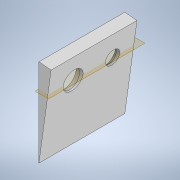
# Autodesk Inventor part: twoPipeCover02
Saved by Autodesk Inventor 2021.1 (Build 251245000, 245)
## iProperties
Created: 2020-07-06
Part Number: twoPipeCover02
Material: Generic
Document SubType Name: Modeling
Designer: robst
Density: 1 g/cm^3
Appearance: Default
Author: robst
Autodesk Inventor part; units mm, degrees
ref_plane "YZ Plane" through (0, 0, 0) normal (1, 0, 0) x (0, 1, 0)
sketch "Sketch1" plane through (0, 0, 0) normal (0, 0, 1) x (1, 0, 0)
  line L0 (0, 0) -> (14.2789, 101.6)
  line L1 (14.2789, 101.6) -> (0, 101.6)
  line L2 (0, 101.6) -> (0, 0)
  dimension "d0" = 101.6
  dimension "d1" = 8
  dimension "d2" = 14.279
  constraints: 6 end point, 1 horizontal, 1 vertical
  measures "d0" distance from line of L0.start L1
  measures "d1" angle of L0 L2
  measures "d2" distance of L0.end L1.end
extrude "MainStructure" add sketch "Sketch1" along normal mid plane 78.74
sketch "Sketch2" plane through (0, 0, 39.37) normal (-1, 0, 0) x (0, 0, 1)
  line L0 (-78.74, 101.6) -> (0, 101.6) projected
  line L1 (-39.37, 101.6) -> (-39.37, 0) construction
  circle A0 centre (-62.23, 73.66) radius 8.255
  circle A1 centre (-16.51, 73.66) radius 11.43
  dimension "d31" = 27.94
  dimension "d32" = 27.94
  dimension "d33" = 22.86
  dimension "d34" = 22.86
  dimension "leftHole" = 22.86
  dimension "rightHole" = 16.51
  constraints: 2 centre point, 2 end point, 1 midpoint, 1 vertical
  measures "d31" distance from line of A0.centre L0
  measures "d32" distance from line of A1.centre L0
  measures "d33" distance from line of A0.centre L1
  measures "d34" distance from line of A1.centre L1
  measures "leftHole" diameter of A1
  measures "rightHole" diameter of A0
extrude "PipeHole" cut sketch "Sketch2" against normal through all
sketch "Sketch6" plane through (0, 0, 0) normal (0, 0, 1) x (1, 0, 0)
  line L0 (0, 101.6) -> (14.2789, 101.6) projected
  line L1 (0, 0) -> (0, 101.6) projected
  line L2 (14.2789, 101.6) -> (0, 0) projected
  line L3 (0, 101.6) -> (14.1055, 100.3659)
  line L4 (14.1055, 100.3659) -> (14.2789, 101.6)
  line L5 (14.2789, 101.6) -> (0, 101.6)
  dimension "d18" = 5
  constraints: 6 end point, 1 collinear, 1 point on line
  measures "d18" angle of L3 L0
extrude "AngleForTopRelief" cut sketch "Sketch6" along normal through all both and the other way through all contours L0 L2 L3
sketch "Sketch7" plane through (0, 0, -39.37) normal (-1, 0, 0) x (0, 0, 1)
  line L0 (0, 0) -> (0, 101.6) construction
  line L1 (0, 50.8) -> (78.74, 50.8) construction
  line L2 (78.74, 0) -> (78.74, 100.3659) construction
  line L3 (0, 0) -> (78.74, 0) projected
  spline S0 degree 2 poles (20.3251, 48.3506) (20.3251, 47.4037) (19.6047, 45.9526) (19.0078, 45.4792) knots 0 0 0 1 2 2 2
  spline S1 degree 2 poles (19.0078, 45.4792) (18.2874, 44.9234) (16.651, 44.45) (15.3542, 44.45) knots 0 0 0 1 2 2 2
  line L4 (15.3542, 44.45) -> (11.711, 44.45)
  line L5 (11.711, 44.45) -> (11.711, 57.15)
  line L6 (11.711, 57.15) -> (15.0764, 57.15)
  spline S2 degree 2 poles (15.0764, 57.15) (16.4349, 57.15) (17.7934, 56.975) (18.4109, 56.6354) knots 0 0 0 1 2 2 2
  spline S3 degree 2 poles (18.4109, 56.6354) (19.1004, 56.2752) (19.7282, 55.0917) (19.7282, 54.2889) knots 0 0 0 1 2 2 2
  spline S4 degree 2 poles (19.7282, 54.2889) (19.7282, 53.3935) (18.7814, 51.9733) (17.9478, 51.5719) knots 0 0 0 1 2 2 2
  line L7 (17.9478, 51.5719) -> (17.9478, 51.5101)
  spline S5 degree 2 poles (17.9478, 51.5101) (19.0798, 51.2014) (20.3251, 49.565) (20.3251, 48.3506) knots 0 0 0 1 2 2 2
  spline S6 degree 2 poles (18.5653, 48.2785) (18.5653, 48.9989) (18.1536, 49.9252) (17.5361, 50.2545) knots 0 0 0 1 2 2 2
  spline S7 degree 2 poles (17.5361, 50.2545) (17.1347, 50.4604) (16.1879, 50.5839) (15.3131, 50.5839) knots 0 0 0 1 2 2 2
  line L8 (15.3131, 50.5839) -> (13.3988, 50.5839)
  line L9 (13.3988, 50.5839) -> (13.3988, 45.8908)
  line L10 (13.3988, 45.8908) -> (14.7676, 45.8908)
  spline S8 degree 2 poles (14.7676, 45.8908) (15.8791, 45.8908) (17.1553, 46.0967) (17.6493, 46.426) knots 0 0 0 1 2 2 2
  spline S9 degree 2 poles (17.6493, 46.426) (18.1227, 46.7656) (18.5653, 47.6096) (18.5653, 48.2785) knots 0 0 0 1 2 2 2
  spline S10 degree 2 poles (17.9683, 54.0522) (17.9683, 54.505) (17.6596, 55.1843) (17.32, 55.3798) knots 0 0 0 1 2 2 2
  spline S11 degree 2 poles (17.32, 55.3798) (16.9083, 55.6062) (15.91, 55.7092) (15.0146, 55.7092) knots 0 0 0 1 2 2 2
  line L11 (15.0146, 55.7092) -> (13.3988, 55.7092)
  line L12 (13.3988, 55.7092) -> (13.3988, 51.9938)
  line L13 (13.3988, 51.9938) -> (15.3131, 51.9938)
  spline S12 degree 2 poles (15.3131, 51.9938) (16.1055, 51.9938) (16.8568, 52.1585) (17.2582, 52.4158) knots 0 0 0 1 2 2 2
  spline S13 degree 2 poles (17.2582, 52.4158) (17.6493, 52.6628) (17.9683, 53.4553) (17.9683, 54.0522) knots 0 0 0 1 2 2 2
  line L14 (26.0885, 44.45) -> (30.3699, 57.15)
  line L15 (30.3699, 57.15) -> (32.4488, 57.15)
  line L16 (32.4488, 57.15) -> (36.7302, 44.45)
  line L17 (36.7302, 44.45) -> (34.9497, 44.45)
  line L18 (34.9497, 44.45) -> (33.797, 48.0006)
  line L19 (33.797, 48.0006) -> (28.9496, 48.0006)
  line L20 (28.9496, 48.0006) -> (27.7969, 44.45)
  line L21 (27.7969, 44.45) -> (26.0885, 44.45)
  line L22 (33.3339, 49.4415) -> (31.3682, 55.421)
  line L23 (31.3682, 55.421) -> (29.4127, 49.4415)
  line L24 (29.4127, 49.4415) -> (33.3339, 49.4415)
  spline S14 degree 2 poles (48.5142, 44.2236) (47.2792, 44.2236) (45.19, 45.0572) (44.4284, 45.8908) knots 0 0 0 1 2 2 2
  spline S15 degree 2 poles (44.4284, 45.8908) (43.6668, 46.7142) (42.8332, 49.1842) (42.8332, 50.7897) knots 0 0 0 1 2 2 2
  spline S16 degree 2 poles (42.8332, 50.7897) (42.8332, 52.3849) (43.6462, 54.752) (44.4181, 55.6268) knots 0 0 0 1 2 2 2
  spline S17 degree 2 poles (44.4181, 55.6268) (45.1797, 56.481) (47.2586, 57.3764) (48.5451, 57.3764) knots 0 0 0 1 2 2 2
  spline S18 degree 2 poles (48.5451, 57.3764) (49.1832, 57.3764) (50.305, 57.1912) (50.7784, 57.0471) knots 0 0 0 1 2 2 2
  spline S19 degree 2 poles (50.7784, 57.0471) (51.1901, 56.9133) (52.0443, 56.5325) (52.4662, 56.3061) knots 0 0 0 1 2 2 2
  line L25 (52.4662, 56.3061) -> (52.4662, 54.2683)
  line L26 (52.4662, 54.2683) -> (52.3324, 54.2683)
  spline S20 degree 2 poles (52.3324, 54.2683) (52.106, 54.4741) (51.4062, 55.0505) (50.9019, 55.3284) knots 0 0 0 1 2 2 2
  spline S21 degree 2 poles (50.9019, 55.3284) (50.4182, 55.5959) (49.2758, 55.9356) (48.5348, 55.9356) knots 0 0 0 1 2 2 2
  spline S22 degree 2 poles (48.5348, 55.9356) (47.7217, 55.9356) (46.2706, 55.2666) (45.7251, 54.6285) knots 0 0 0 1 2 2 2
  spline S23 degree 2 poles (45.7251, 54.6285) (45.19, 53.9801) (44.5931, 52.0144) (44.5931, 50.7897) knots 0 0 0 1 2 2 2
  spline S24 degree 2 poles (44.5931, 50.7897) (44.5931, 49.4827) (45.2209, 47.5993) (45.7663, 46.9509) knots 0 0 0 1 2 2 2
  spline S25 degree 2 poles (45.7663, 46.9509) (46.3015, 46.3231) (47.732, 45.685) (48.5348, 45.685) knots 0 0 0 1 2 2 2
  spline S26 degree 2 poles (48.5348, 45.685) (49.2655, 45.685) (50.5108, 46.0452) (50.9945, 46.3128) knots 0 0 0 1 2 2 2
  spline S27 degree 2 poles (50.9945, 46.3128) (51.4576, 46.5804) (52.1472, 47.1361) (52.3427, 47.3317) knots 0 0 0 1 2 2 2
  line L27 (52.3427, 47.3317) -> (52.4662, 47.3317)
  line L28 (52.4662, 47.3317) -> (52.4662, 45.3145)
  spline S28 degree 2 poles (52.4662, 45.3145) (52.0443, 45.119) (51.3033, 44.7588) (50.7784, 44.5941) knots 0 0 0 1 2 2 2
  spline S29 degree 2 poles (50.7784, 44.5941) (50.2226, 44.4088) (49.2758, 44.2236) (48.5142, 44.2236) knots 0 0 0 1 2 2 2
  line L29 (68.758, 44.45) -> (66.5659, 44.45)
  line L30 (66.5659, 44.45) -> (61.9243, 50.3575)
  line L31 (61.9243, 50.3575) -> (61.1833, 49.5238)
  line L32 (61.1833, 49.5238) -> (61.1833, 44.45)
  line L33 (61.1833, 44.45) -> (59.4955, 44.45)
  line L34 (59.4955, 44.45) -> (59.4955, 57.15)
  line L35 (59.4955, 57.15) -> (61.1833, 57.15)
  line L36 (61.1833, 57.15) -> (61.1833, 51.3146)
  line L37 (61.1833, 51.3146) -> (66.3909, 57.15)
  line L38 (66.3909, 57.15) -> (68.4493, 57.15)
  line L39 (68.4493, 57.15) -> (63.1902, 51.4793)
  line L40 (63.1902, 51.4793) -> (68.758, 44.45)
  point P0 (39.37, 0)
  dimension "largeTextLine" = 50.8
  constraints: 2 end point, 2 horizontal, 1 midpoint, 1 point on line
  measures "largeTextLine" distance between parallel lines of L3 L1
extrude "TextForBack" cut sketch "Sketch7" against normal blind 1.27
sketch "Sketch8" plane through (0, 0, -39.37) normal (-1, 0, 0) x (0, 0, 1)
  arc A0 (24.765, 73.66) -> (24.765, 73.66) centre (16.51, 73.66) ccw projected
  circle A1 centre (62.23, 73.66) radius 11.43 projected
  circle A2 centre (16.51, 73.66) radius 14.2875
  circle A3 centre (62.23, 73.66) radius 13.97
  point P0 (39.37, 0)
  dimension "rightHoleRelief" = 28.575
  dimension "leftHoleRelief" = 27.94
  constraints: 2 centre point, 2 coincident
  measures "rightHoleRelief" diameter of A2
  measures "leftHoleRelief" diameter of A3
extrude "ReliefForHole" cut sketch "Sketch8" against normal blind 6.35 contours A0 | A2 | A3
ref_plane "Work Plane1" through (0, 0, 22.86) normal (0, 0, 1) x (1, 0, 0)
ref_plane "Work Plane2" through (0, 0, -22.86) normal (0, 0, 1) x (1, 0, 0)
sketch "Sketch9" plane through (0, 0, -39.37) normal (-1, 0, 0) x (0, 0, 1)
  line L0 (0, 100.3659) -> (0, 0) construction
  line L1 (0, 93.98) -> (78.74, 93.98) construction
  line L2 (78.74, 0) -> (78.74, 100.3659) construction
  line L3 (0, 101.6) -> (78.74, 101.6) construction
  spline S0 degree 2 poles (21.9449, 92.4124) (21.9449, 91.8064) (21.4838, 90.8777) (21.1018, 90.5747) knots 0 0 0 1 2 2 2
  spline S1 degree 2 poles (21.1018, 90.5747) (20.6407, 90.219) (19.5934, 89.916) (18.7635, 89.916) knots 0 0 0 1 2 2 2
  line L4 (18.7635, 89.916) -> (16.4318, 89.916)
  line L5 (16.4318, 89.916) -> (16.4318, 98.044)
  line L6 (16.4318, 98.044) -> (18.5856, 98.044)
  spline S2 degree 2 poles (18.5856, 98.044) (19.4551, 98.044) (20.3245, 97.932) (20.7197, 97.7147) knots 0 0 0 1 2 2 2
  spline S3 degree 2 poles (20.7197, 97.7147) (21.161, 97.4841) (21.5628, 96.7267) (21.5628, 96.2129) knots 0 0 0 1 2 2 2
  spline S4 degree 2 poles (21.5628, 96.2129) (21.5628, 95.6399) (20.9569, 94.7309) (20.4233, 94.474) knots 0 0 0 1 2 2 2
  line L7 (20.4233, 94.474) -> (20.4233, 94.4345)
  spline S5 degree 2 poles (20.4233, 94.4345) (21.1479, 94.2369) (21.9449, 93.1896) (21.9449, 92.4124) knots 0 0 0 1 2 2 2
  spline S6 degree 2 poles (20.8185, 92.3663) (20.8185, 92.8273) (20.5551, 93.4201) (20.1599, 93.6309) knots 0 0 0 1 2 2 2
  spline S7 degree 2 poles (20.1599, 93.6309) (19.903, 93.7626) (19.297, 93.8417) (18.7371, 93.8417) knots 0 0 0 1 2 2 2
  line L8 (18.7371, 93.8417) -> (17.512, 93.8417)
  line L9 (17.512, 93.8417) -> (17.512, 90.8381)
  line L10 (17.512, 90.8381) -> (18.388, 90.8381)
  spline S8 degree 2 poles (18.388, 90.8381) (19.0994, 90.8381) (19.9162, 90.9699) (20.2323, 91.1806) knots 0 0 0 1 2 2 2
  spline S9 degree 2 poles (20.2323, 91.1806) (20.5353, 91.398) (20.8185, 91.9381) (20.8185, 92.3663) knots 0 0 0 1 2 2 2
  spline S10 degree 2 poles (20.4365, 96.0614) (20.4365, 96.3512) (20.2389, 96.7859) (20.0215, 96.9111) knots 0 0 0 1 2 2 2
  spline S11 degree 2 poles (20.0215, 96.9111) (19.7581, 97.056) (19.1192, 97.1219) (18.5461, 97.1219) knots 0 0 0 1 2 2 2
  line L11 (18.5461, 97.1219) -> (17.512, 97.1219)
  line L12 (17.512, 97.1219) -> (17.512, 94.7441)
  line L13 (17.512, 94.7441) -> (18.7371, 94.7441)
  spline S12 degree 2 poles (18.7371, 94.7441) (19.2443, 94.7441) (19.7251, 94.8494) (19.982, 95.0141) knots 0 0 0 1 2 2 2
  spline S13 degree 2 poles (19.982, 95.0141) (20.2323, 95.1722) (20.4365, 95.6794) (20.4365, 96.0614) knots 0 0 0 1 2 2 2
  line L14 (29.1244, 89.916) -> (31.8644, 98.044)
  line L15 (31.8644, 98.044) -> (33.195, 98.044)
  line L16 (33.195, 98.044) -> (35.935, 89.916)
  line L17 (35.935, 89.916) -> (34.7955, 89.916)
  line L18 (34.7955, 89.916) -> (34.0578, 92.1884)
  line L19 (34.0578, 92.1884) -> (30.9555, 92.1884)
  line L20 (30.9555, 92.1884) -> (30.2178, 89.916)
  line L21 (30.2178, 89.916) -> (29.1244, 89.916)
  line L22 (33.7614, 93.1106) -> (32.5034, 96.9374)
  line L23 (32.5034, 96.9374) -> (31.2519, 93.1106)
  line L24 (31.2519, 93.1106) -> (33.7614, 93.1106)
  spline S14 degree 2 poles (46.9678, 89.7711) (46.1774, 89.7711) (44.8403, 90.3046) (44.3528, 90.8381) knots 0 0 0 1 2 2 2
  spline S15 degree 2 poles (44.3528, 90.8381) (43.8654, 91.3651) (43.3319, 92.9459) (43.3319, 93.9734) knots 0 0 0 1 2 2 2
  spline S16 degree 2 poles (43.3319, 93.9734) (43.3319, 94.9944) (43.8523, 96.5093) (44.3463, 97.0692) knots 0 0 0 1 2 2 2
  spline S17 degree 2 poles (44.3463, 97.0692) (44.8337, 97.6159) (46.1642, 98.1889) (46.9875, 98.1889) knots 0 0 0 1 2 2 2
  spline S18 degree 2 poles (46.9875, 98.1889) (47.3959, 98.1889) (48.1139, 98.0703) (48.4168, 97.9781) knots 0 0 0 1 2 2 2
  spline S19 degree 2 poles (48.4168, 97.9781) (48.6803, 97.8925) (49.227, 97.6488) (49.4971, 97.5039) knots 0 0 0 1 2 2 2
  line L25 (49.4971, 97.5039) -> (49.4971, 96.1997)
  line L26 (49.4971, 96.1997) -> (49.4114, 96.1997)
  spline S20 degree 2 poles (49.4114, 96.1997) (49.2665, 96.3315) (48.8186, 96.7003) (48.4959, 96.8782) knots 0 0 0 1 2 2 2
  spline S21 degree 2 poles (48.4959, 96.8782) (48.1863, 97.0494) (47.4552, 97.2668) (46.9809, 97.2668) knots 0 0 0 1 2 2 2
  spline S22 degree 2 poles (46.9809, 97.2668) (46.4606, 97.2668) (45.5319, 96.8386) (45.1828, 96.4303) knots 0 0 0 1 2 2 2
  spline S23 degree 2 poles (45.1828, 96.4303) (44.8403, 96.0153) (44.4582, 94.7572) (44.4582, 93.9734) knots 0 0 0 1 2 2 2
  spline S24 degree 2 poles (44.4582, 93.9734) (44.4582, 93.1369) (44.86, 91.9315) (45.2091, 91.5166) knots 0 0 0 1 2 2 2
  spline S25 degree 2 poles (45.2091, 91.5166) (45.5516, 91.1148) (46.4672, 90.7064) (46.9809, 90.7064) knots 0 0 0 1 2 2 2
  spline S26 degree 2 poles (46.9809, 90.7064) (47.4486, 90.7064) (48.2456, 90.9369) (48.5552, 91.1082) knots 0 0 0 1 2 2 2
  spline S27 degree 2 poles (48.5552, 91.1082) (48.8516, 91.2794) (49.2929, 91.6351) (49.418, 91.7603) knots 0 0 0 1 2 2 2
  line L27 (49.418, 91.7603) -> (49.4971, 91.7603)
  line L28 (49.4971, 91.7603) -> (49.4971, 90.4693)
  spline S28 degree 2 poles (49.4971, 90.4693) (49.227, 90.3441) (48.7528, 90.1136) (48.4168, 90.0082) knots 0 0 0 1 2 2 2
  spline S29 degree 2 poles (48.4168, 90.0082) (48.0612, 89.8897) (47.4552, 89.7711) (46.9678, 89.7711) knots 0 0 0 1 2 2 2
  line L29 (63.4148, 89.916) -> (62.0118, 89.916)
  line L30 (62.0118, 89.916) -> (59.0412, 93.6968)
  line L31 (59.0412, 93.6968) -> (58.567, 93.1632)
  line L32 (58.567, 93.1632) -> (58.567, 89.916)
  line L33 (58.567, 89.916) -> (57.4867, 89.916)
  line L34 (57.4867, 89.916) -> (57.4867, 98.044)
  line L35 (57.4867, 98.044) -> (58.567, 98.044)
  line L36 (58.567, 98.044) -> (58.567, 94.3093)
  line L37 (58.567, 94.3093) -> (61.8998, 98.044)
  line L38 (61.8998, 98.044) -> (63.2172, 98.044)
  line L39 (63.2172, 98.044) -> (59.8514, 94.4147)
  line L40 (59.8514, 94.4147) -> (63.4148, 89.916)
  point P0 (39.37, 0)
  dimension "d41" = 7.62
  constraints: 2 end point, 2 horizontal, 2 point on line
  measures "d41" distance between parallel lines of L1 L3
extrude "SmallTextForBack" cut sketch "Sketch9" against normal blind 1.27
ref_plane "Work Plane3" through (0, 101.6, 39.37) normal (0, 1, 0) x (-1, 0, 0)
ref_plane "Work Plane4" through (0, 73.66, 0) normal (0, 1, 0) x (-1, 0, 0)
sketch "Sketch11" plane through (0, 0, -39.37) normal (-1, 0, 0) x (0, 0, 1)
  line L0 (0, 100.3659) -> (0, 0) construction
  line L1 (0, 31.75) -> (78.74, 31.75) construction
  line L2 (78.74, 0) -> (78.74, 100.3659) construction
  line L3 (0, 0) -> (78.74, 0) construction
  spline S0 degree 2 poles (4.6076, 27.8288) (3.8234, 27.8288) (2.9403, 28.7242) (2.9403, 29.6937) knots 0 0 0 1 2 2 2
  line L4 (2.9403, 29.6937) -> (2.9403, 32.8615)
  line L5 (2.9403, 32.8615) -> (2.292, 32.8615)
  line L6 (2.292, 32.8615) -> (2.292, 33.6581)
  line L7 (2.292, 33.6581) -> (2.9403, 33.6581)
  line L8 (2.9403, 33.6581) -> (2.9403, 35.3006)
  line L9 (2.9403, 35.3006) -> (3.9037, 35.3006)
  line L10 (3.9037, 35.3006) -> (3.9037, 33.6581)
  line L11 (3.9037, 33.6581) -> (5.6759, 33.6581)
  line L12 (5.6759, 33.6581) -> (5.6759, 32.8615)
  line L13 (5.6759, 32.8615) -> (3.9037, 32.8615)
  line L14 (3.9037, 32.8615) -> (3.9037, 30.1383)
  spline S1 degree 2 poles (3.9037, 30.1383) (3.9037, 29.7061) (3.9345, 29.2306) (4.0395, 29.0268) knots 0 0 0 1 2 2 2
  spline S2 degree 2 poles (4.0395, 29.0268) (4.126, 28.8477) (4.515, 28.6687) (4.8484, 28.6687) knots 0 0 0 1 2 2 2
  spline S3 degree 2 poles (4.8484, 28.6687) (5.0831, 28.6687) (5.5215, 28.8107) (5.6203, 28.8539) knots 0 0 0 1 2 2 2
  line L15 (5.6203, 28.8539) -> (5.6759, 28.8539)
  line L16 (5.6759, 28.8539) -> (5.6759, 27.9894)
  spline S4 degree 2 poles (5.6759, 27.9894) (5.4042, 27.9153) (4.8484, 27.8288) (4.6076, 27.8288) knots 0 0 0 1 2 2 2
  line L17 (13.3144, 33.6581) -> (11.8633, 27.94)
  line L18 (11.8633, 27.94) -> (10.9741, 27.94)
  line L19 (10.9741, 27.94) -> (9.5785, 32.349)
  line L20 (9.5785, 32.349) -> (8.1891, 27.94)
  line L21 (8.1891, 27.94) -> (7.3061, 27.94)
  line L22 (7.3061, 27.94) -> (5.8426, 33.6581)
  line L23 (5.8426, 33.6581) -> (6.843, 33.6581)
  line L24 (6.843, 33.6581) -> (7.8557, 29.2306)
  line L25 (7.8557, 29.2306) -> (9.208, 33.6581)
  line L26 (9.208, 33.6581) -> (10.0046, 33.6581)
  line L27 (10.0046, 33.6581) -> (11.394, 29.2306)
  line L28 (11.394, 29.2306) -> (12.3449, 33.6581)
  line L29 (12.3449, 33.6581) -> (13.3144, 33.6581)
  spline S5 degree 2 poles (18.8596, 30.799) (18.8596, 29.3541) (17.4702, 27.7794) (16.3093, 27.7794) knots 0 0 0 1 2 2 2
  spline S6 degree 2 poles (16.3093, 27.7794) (15.1175, 27.7794) (13.7528, 29.4035) (13.7528, 30.799) knots 0 0 0 1 2 2 2
  spline S7 degree 2 poles (13.7528, 30.799) (13.7528, 32.2317) (15.1608, 33.8186) (16.3093, 33.8186) knots 0 0 0 1 2 2 2
  spline S8 degree 2 poles (16.3093, 33.8186) (17.4702, 33.8186) (18.8596, 32.2378) (18.8596, 30.799) knots 0 0 0 1 2 2 2
  spline S9 degree 2 poles (17.8654, 30.799) (17.8654, 31.9106) (17.0565, 32.9912) (16.3093, 32.9912) knots 0 0 0 1 2 2 2
  spline S10 degree 2 poles (16.3093, 32.9912) (15.5621, 32.9912) (14.747, 31.9106) (14.747, 30.799) knots 0 0 0 1 2 2 2
  spline S11 degree 2 poles (14.747, 30.799) (14.747, 29.7184) (15.5621, 28.6069) (16.3093, 28.6069) knots 0 0 0 1 2 2 2
  spline S12 degree 2 poles (16.3093, 28.6069) (17.0503, 28.6069) (17.8654, 29.6999) (17.8654, 30.799) knots 0 0 0 1 2 2 2
  spline S13 degree 2 poles (24.7382, 33.2629) (24.7382, 32.7689) (24.3863, 31.8797) (24.0713, 31.5709) knots 0 0 0 1 2 2 2
  spline S14 degree 2 poles (24.0713, 31.5709) (23.6761, 31.1819) (22.6079, 30.7805) (21.7927, 30.7805) knots 0 0 0 1 2 2 2
  line L30 (21.7927, 30.7805) -> (20.9344, 30.7805)
  line L31 (20.9344, 30.7805) -> (20.9344, 27.94)
  line L32 (20.9344, 27.94) -> (19.9217, 27.94)
  line L33 (19.9217, 27.94) -> (19.9217, 35.56)
  line L34 (19.9217, 35.56) -> (21.836, 35.56)
  spline S15 degree 2 poles (21.836, 35.56) (22.5152, 35.56) (23.4662, 35.3377) (23.8305, 35.0845) knots 0 0 0 1 2 2 2
  spline S16 degree 2 poles (23.8305, 35.0845) (24.2566, 34.7943) (24.7382, 33.8989) (24.7382, 33.2629) knots 0 0 0 1 2 2 2
  spline S17 degree 2 poles (23.6823, 33.232) (23.6823, 33.6272) (23.4106, 34.2077) (23.1327, 34.3929) knots 0 0 0 1 2 2 2
  spline S18 degree 2 poles (23.1327, 34.3929) (22.8919, 34.5535) (22.2497, 34.6831) (21.7742, 34.6831) knots 0 0 0 1 2 2 2
  line L35 (21.7742, 34.6831) -> (20.9344, 34.6831)
  line L36 (20.9344, 34.6831) -> (20.9344, 31.645)
  line L37 (20.9344, 31.645) -> (21.626, 31.645)
  spline S19 degree 2 poles (21.626, 31.645) (22.2435, 31.645) (23.0031, 31.8426) (23.2501, 32.102) knots 0 0 0 1 2 2 2
  spline S20 degree 2 poles (23.2501, 32.102) (23.4785, 32.3305) (23.6823, 32.8677) (23.6823, 33.232) knots 0 0 0 1 2 2 2
  line L38 (26.6093, 27.94) -> (25.646, 27.94)
  line L39 (25.646, 27.94) -> (25.646, 33.6581)
  line L40 (25.646, 33.6581) -> (26.6093, 33.6581)
  line L41 (26.6093, 33.6581) -> (26.6093, 27.94)
  line L42 (26.6772, 34.609) -> (25.5842, 34.609)
  line L43 (25.5842, 34.609) -> (25.5842, 35.6094)
  line L44 (25.5842, 35.6094) -> (26.6772, 35.6094)
  line L45 (26.6772, 35.6094) -> (26.6772, 34.609)
  spline S21 degree 2 poles (32.8152, 30.9534) (32.8152, 29.5208) (31.4505, 27.8288) (30.4069, 27.8288) knots 0 0 0 1 2 2 2
  spline S22 degree 2 poles (30.4069, 27.8288) (29.9808, 27.8288) (29.3263, 28.0265) (28.9867, 28.2302) knots 0 0 0 1 2 2 2
  line L46 (28.9867, 28.2302) -> (28.9867, 25.8343)
  line L47 (28.9867, 25.8343) -> (28.0234, 25.8343)
  line L48 (28.0234, 25.8343) -> (28.0234, 33.6581)
  line L49 (28.0234, 33.6581) -> (28.9867, 33.6581)
  line L50 (28.9867, 33.6581) -> (28.9867, 33.0591)
  spline S23 degree 2 poles (28.9867, 33.0591) (29.3448, 33.3864) (30.2217, 33.8186) (30.7342, 33.8186) knots 0 0 0 1 2 2 2
  spline S24 degree 2 poles (30.7342, 33.8186) (31.716, 33.8186) (32.8152, 32.2625) (32.8152, 30.9534) knots 0 0 0 1 2 2 2
  spline S25 degree 2 poles (31.821, 30.8423) (31.821, 31.8241) (31.1973, 32.9047) (30.4996, 32.9047) knots 0 0 0 1 2 2 2
  spline S26 degree 2 poles (30.4996, 32.9047) (30.092, 32.9047) (29.3263, 32.5404) (28.9867, 32.2564) knots 0 0 0 1 2 2 2
  line L51 (28.9867, 32.2564) -> (28.9867, 29.0083)
  spline S27 degree 2 poles (28.9867, 29.0083) (29.3633, 28.8292) (29.9006, 28.6934) (30.2464, 28.6934) knots 0 0 0 1 2 2 2
  spline S28 degree 2 poles (30.2464, 28.6934) (30.9936, 28.6934) (31.821, 29.7925) (31.821, 30.8423) knots 0 0 0 1 2 2 2
  spline S29 degree 2 poles (36.2979, 27.8103) (34.9271, 27.8103) (33.4203, 29.3479) (33.4203, 30.7682) knots 0 0 0 1 2 2 2
  spline S30 degree 2 poles (33.4203, 30.7682) (33.4203, 32.1637) (34.8838, 33.8186) (36.0633, 33.8186) knots 0 0 0 1 2 2 2
  spline S31 degree 2 poles (36.0633, 33.8186) (36.5943, 33.8186) (37.4156, 33.5099) (37.7182, 33.1826) knots 0 0 0 1 2 2 2
  spline S32 degree 2 poles (37.7182, 33.1826) (38.0269, 32.8553) (38.3542, 31.9106) (38.3542, 31.2251) knots 0 0 0 1 2 2 2
  line L52 (38.3542, 31.2251) -> (38.3542, 30.7002)
  line L53 (38.3542, 30.7002) -> (34.396, 30.7002)
  spline S33 degree 2 poles (34.396, 30.7002) (34.396, 29.7061) (35.3964, 28.6501) (36.2856, 28.6501) knots 0 0 0 1 2 2 2
  spline S34 degree 2 poles (36.2856, 28.6501) (36.6005, 28.6501) (37.2118, 28.7922) (37.4588, 28.9033) knots 0 0 0 1 2 2 2
  spline S35 degree 2 poles (37.4588, 28.9033) (37.7182, 29.0268) (38.0763, 29.2429) (38.1937, 29.3417) knots 0 0 0 1 2 2 2
  line L54 (38.1937, 29.3417) -> (38.2492, 29.3417)
  line L55 (38.2492, 29.3417) -> (38.2492, 28.292)
  spline S36 degree 2 poles (38.2492, 28.292) (38.0825, 28.2241) (37.5761, 28.0265) (37.3785, 27.9709) knots 0 0 0 1 2 2 2
  spline S37 degree 2 poles (37.3785, 27.9709) (37.1007, 27.8906) (36.6437, 27.8103) (36.2979, 27.8103) knots 0 0 0 1 2 2 2
  spline S38 degree 2 poles (37.4156, 31.4351) (37.4032, 31.8241) (37.2427, 32.3922) (37.0883, 32.5836) knots 0 0 0 1 2 2 2
  spline S39 degree 2 poles (37.0883, 32.5836) (36.9216, 32.7998) (36.3967, 33.0282) (36.0077, 33.0282) knots 0 0 0 1 2 2 2
  spline S40 degree 2 poles (36.0077, 33.0282) (35.6248, 33.0282) (35.0876, 32.7998) (34.8653, 32.5775) knots 0 0 0 1 2 2 2
  spline S41 degree 2 poles (34.8653, 32.5775) (34.6492, 32.349) (34.4269, 31.7994) (34.396, 31.4351) knots 0 0 0 1 2 2 2
  line L56 (34.396, 31.4351) -> (37.4156, 31.4351)
  spline S42 degree 2 poles (42.3803, 27.8041) (41.6393, 27.8041) (40.3858, 28.3043) (39.9288, 28.8045) knots 0 0 0 1 2 2 2
  spline S43 degree 2 poles (39.9288, 28.8045) (39.4719, 29.2985) (38.9717, 30.7805) (38.9717, 31.7438) knots 0 0 0 1 2 2 2
  spline S44 degree 2 poles (38.9717, 31.7438) (38.9717, 32.701) (39.4595, 34.1212) (39.9227, 34.6461) knots 0 0 0 1 2 2 2
  spline S45 degree 2 poles (39.9227, 34.6461) (40.3796, 35.1586) (41.627, 35.6959) (42.3989, 35.6959) knots 0 0 0 1 2 2 2
  spline S46 degree 2 poles (42.3989, 35.6959) (42.7817, 35.6959) (43.4548, 35.5847) (43.7388, 35.4982) knots 0 0 0 1 2 2 2
  spline S47 degree 2 poles (43.7388, 35.4982) (43.9858, 35.418) (44.4984, 35.1895) (44.7515, 35.0536) knots 0 0 0 1 2 2 2
  line L57 (44.7515, 35.0536) -> (44.7515, 33.831)
  line L58 (44.7515, 33.831) -> (44.6713, 33.831)
  spline S48 degree 2 poles (44.6713, 33.831) (44.5354, 33.9545) (44.1155, 34.3003) (43.8129, 34.467) knots 0 0 0 1 2 2 2
  spline S49 degree 2 poles (43.8129, 34.467) (43.5227, 34.6276) (42.8373, 34.8313) (42.3927, 34.8313) knots 0 0 0 1 2 2 2
  spline S50 degree 2 poles (42.3927, 34.8313) (41.9049, 34.8313) (41.0342, 34.43) (40.7069, 34.0471) knots 0 0 0 1 2 2 2
  spline S51 degree 2 poles (40.7069, 34.0471) (40.3858, 33.6581) (40.0276, 32.4787) (40.0276, 31.7438) knots 0 0 0 1 2 2 2
  spline S52 degree 2 poles (40.0276, 31.7438) (40.0276, 30.9596) (40.4043, 29.8296) (40.7316, 29.4405) knots 0 0 0 1 2 2 2
  spline S53 degree 2 poles (40.7316, 29.4405) (41.0527, 29.0639) (41.911, 28.681) (42.3927, 28.681) knots 0 0 0 1 2 2 2
  spline S54 degree 2 poles (42.3927, 28.681) (42.8311, 28.681) (43.5783, 28.8971) (43.8685, 29.0577) knots 0 0 0 1 2 2 2
  spline S55 degree 2 poles (43.8685, 29.0577) (44.1464, 29.2182) (44.5601, 29.5517) (44.6774, 29.669) knots 0 0 0 1 2 2 2
  line L59 (44.6774, 29.669) -> (44.7515, 29.669)
  line L60 (44.7515, 29.669) -> (44.7515, 28.4587)
  spline S56 degree 2 poles (44.7515, 28.4587) (44.4984, 28.3414) (44.0538, 28.1253) (43.7388, 28.0265) knots 0 0 0 1 2 2 2
  spline S57 degree 2 poles (43.7388, 28.0265) (43.4054, 27.9153) (42.8373, 27.8041) (42.3803, 27.8041) knots 0 0 0 1 2 2 2
  spline S58 degree 2 poles (50.3214, 30.799) (50.3214, 29.3541) (48.932, 27.7794) (47.7711, 27.7794) knots 0 0 0 1 2 2 2
  spline S59 degree 2 poles (47.7711, 27.7794) (46.5794, 27.7794) (45.2147, 29.4035) (45.2147, 30.799) knots 0 0 0 1 2 2 2
  spline S60 degree 2 poles (45.2147, 30.799) (45.2147, 32.2317) (46.6226, 33.8186) (47.7711, 33.8186) knots 0 0 0 1 2 2 2
  spline S61 degree 2 poles (47.7711, 33.8186) (48.932, 33.8186) (50.3214, 32.2378) (50.3214, 30.799) knots 0 0 0 1 2 2 2
  spline S62 degree 2 poles (49.3273, 30.799) (49.3273, 31.9106) (48.5183, 32.9912) (47.7711, 32.9912) knots 0 0 0 1 2 2 2
  spline S63 degree 2 poles (47.7711, 32.9912) (47.024, 32.9912) (46.2089, 31.9106) (46.2089, 30.799) knots 0 0 0 1 2 2 2
  spline S64 degree 2 poles (46.2089, 30.799) (46.2089, 29.7184) (47.024, 28.6069) (47.7711, 28.6069) knots 0 0 0 1 2 2 2
  spline S65 degree 2 poles (47.7711, 28.6069) (48.5121, 28.6069) (49.3273, 29.6999) (49.3273, 30.799) knots 0 0 0 1 2 2 2
  line L61 (55.7987, 33.6581) -> (53.6436, 27.94)
  line L62 (53.6436, 27.94) -> (52.7791, 27.94)
  line L63 (52.7791, 27.94) -> (50.6425, 33.6581)
  line L64 (50.6425, 33.6581) -> (51.6861, 33.6581)
  line L65 (51.6861, 33.6581) -> (53.2484, 29.2553)
  line L66 (53.2484, 29.2553) -> (54.7983, 33.6581)
  line L67 (54.7983, 33.6581) -> (55.7987, 33.6581)
  spline S66 degree 2 poles (59.0097, 27.8103) (57.6389, 27.8103) (56.1321, 29.3479) (56.1321, 30.7682) knots 0 0 0 1 2 2 2
  spline S67 degree 2 poles (56.1321, 30.7682) (56.1321, 32.1637) (57.5956, 33.8186) (58.7751, 33.8186) knots 0 0 0 1 2 2 2
  spline S68 degree 2 poles (58.7751, 33.8186) (59.3061, 33.8186) (60.1274, 33.5099) (60.43, 33.1826) knots 0 0 0 1 2 2 2
  spline S69 degree 2 poles (60.43, 33.1826) (60.7387, 32.8553) (61.066, 31.9106) (61.066, 31.2251) knots 0 0 0 1 2 2 2
  line L68 (61.066, 31.2251) -> (61.066, 30.7002)
  line L69 (61.066, 30.7002) -> (57.1078, 30.7002)
  spline S70 degree 2 poles (57.1078, 30.7002) (57.1078, 29.7061) (58.1082, 28.6501) (58.9974, 28.6501) knots 0 0 0 1 2 2 2
  spline S71 degree 2 poles (58.9974, 28.6501) (59.3123, 28.6501) (59.9236, 28.7922) (60.1706, 28.9033) knots 0 0 0 1 2 2 2
  spline S72 degree 2 poles (60.1706, 28.9033) (60.43, 29.0268) (60.7881, 29.2429) (60.9055, 29.3417) knots 0 0 0 1 2 2 2
  line L70 (60.9055, 29.3417) -> (60.961, 29.3417)
  line L71 (60.961, 29.3417) -> (60.961, 28.292)
  spline S73 degree 2 poles (60.961, 28.292) (60.7943, 28.2241) (60.2879, 28.0265) (60.0903, 27.9709) knots 0 0 0 1 2 2 2
  spline S74 degree 2 poles (60.0903, 27.9709) (59.8125, 27.8906) (59.3555, 27.8103) (59.0097, 27.8103) knots 0 0 0 1 2 2 2
  spline S75 degree 2 poles (60.1274, 31.4351) (60.115, 31.8241) (59.9545, 32.3922) (59.8001, 32.5836) knots 0 0 0 1 2 2 2
  spline S76 degree 2 poles (59.8001, 32.5836) (59.6334, 32.7998) (59.1085, 33.0282) (58.7195, 33.0282) knots 0 0 0 1 2 2 2
  spline S77 degree 2 poles (58.7195, 33.0282) (58.3366, 33.0282) (57.7994, 32.7998) (57.5771, 32.5775) knots 0 0 0 1 2 2 2
  spline S78 degree 2 poles (57.5771, 32.5775) (57.361, 32.349) (57.1387, 31.7994) (57.1078, 31.4351) knots 0 0 0 1 2 2 2
  line L72 (57.1078, 31.4351) -> (60.1274, 31.4351)
  line L73 (65.0736, 32.6269) -> (65.0242, 32.6269)
  spline S79 degree 2 poles (65.0242, 32.6269) (64.9131, 32.6577) (64.6722, 32.6701) (64.5055, 32.6701) knots 0 0 0 1 2 2 2
  spline S80 degree 2 poles (64.5055, 32.6701) (64.1165, 32.6701) (63.3508, 32.3305) (63.005, 31.997) knots 0 0 0 1 2 2 2
  line L74 (63.005, 31.997) -> (63.005, 27.94)
  line L75 (63.005, 27.94) -> (62.0417, 27.94)
  line L76 (62.0417, 27.94) -> (62.0417, 33.6581)
  line L77 (62.0417, 33.6581) -> (63.005, 33.6581)
  line L78 (63.005, 33.6581) -> (63.005, 32.8059)
  spline S81 degree 2 poles (63.005, 32.8059) (63.5298, 33.2752) (64.3141, 33.6581) (64.6846, 33.6581) knots 0 0 0 1 2 2 2
  spline S82 degree 2 poles (64.6846, 33.6581) (64.8328, 33.6581) (64.981, 33.6457) (65.0736, 33.6272) knots 0 0 0 1 2 2 2
  line L79 (65.0736, 33.6272) -> (65.0736, 32.6269)
  spline S83 degree 2 poles (70.4212, 31.75) (70.4212, 29.6999) (69.2294, 27.7794) (67.9882, 27.7794) knots 0 0 0 1 2 2 2
  spline S84 degree 2 poles (67.9882, 27.7794) (66.7285, 27.7794) (65.5491, 29.7369) (65.5491, 31.7438) knots 0 0 0 1 2 2 2
  spline S85 degree 2 poles (65.5491, 31.7438) (65.5491, 33.8063) (66.7409, 35.7144) (67.9882, 35.7144) knots 0 0 0 1 2 2 2
  spline S86 degree 2 poles (67.9882, 35.7144) (69.2418, 35.7144) (70.4212, 33.7384) (70.4212, 31.75) knots 0 0 0 1 2 2 2
  spline S87 degree 2 poles (69.1121, 29.4282) (69.2603, 29.8049) (69.3838, 30.9658) (69.3838, 31.75) knots 0 0 0 1 2 2 2
  spline S88 degree 2 poles (69.3838, 31.75) (69.3838, 32.5342) (69.2603, 33.689) (69.1059, 34.078) knots 0 0 0 1 2 2 2
  spline S89 degree 2 poles (69.1059, 34.078) (68.9515, 34.467) (68.4143, 34.8684) (67.9882, 34.8684) knots 0 0 0 1 2 2 2
  spline S90 degree 2 poles (67.9882, 34.8684) (67.5621, 34.8684) (67.0126, 34.467) (66.852, 34.0656) knots 0 0 0 1 2 2 2
  spline S91 degree 2 poles (66.852, 34.0656) (66.6976, 33.6766) (66.5865, 32.491) (66.5865, 31.7438) knots 0 0 0 1 2 2 2
  spline S92 degree 2 poles (66.5865, 31.7438) (66.5865, 30.9411) (66.6853, 29.8666) (66.8458, 29.4467) knots 0 0 0 1 2 2 2
  spline S93 degree 2 poles (66.8458, 29.4467) (66.994, 29.0515) (67.5436, 28.6254) (67.9882, 28.6254) knots 0 0 0 1 2 2 2
  spline S94 degree 2 poles (67.9882, 28.6254) (68.4081, 28.6254) (68.9577, 29.0268) (69.1121, 29.4282) knots 0 0 0 1 2 2 2
  line L80 (76.0961, 27.94) -> (71.3968, 27.94)
  line L81 (71.3968, 27.94) -> (71.3968, 29.0206)
  spline S95 degree 2 poles (71.3968, 29.0206) (71.9032, 29.4961) (72.8048, 30.3791) (73.237, 30.8546) knots 0 0 0 1 2 2 2
  spline S96 degree 2 poles (73.237, 30.8546) (74.1077, 31.8118) (74.7437, 32.9603) (74.7437, 33.5716) knots 0 0 0 1 2 2 2
  spline S97 degree 2 poles (74.7437, 33.5716) (74.7437, 33.8927) (74.5461, 34.3744) (74.367, 34.5288) knots 0 0 0 1 2 2 2
  spline S98 degree 2 poles (74.367, 34.5288) (74.188, 34.6831) (73.7187, 34.8375) (73.4346, 34.8375) knots 0 0 0 1 2 2 2
  spline S99 degree 2 poles (73.4346, 34.8375) (73.1629, 34.8375) (72.6072, 34.7017) (72.354, 34.5967) knots 0 0 0 1 2 2 2
  spline S100 degree 2 poles (72.354, 34.5967) (72.1379, 34.5102) (71.7365, 34.2632) (71.613, 34.1768) knots 0 0 0 1 2 2 2
  line L82 (71.613, 34.1768) -> (71.5574, 34.1768)
  line L83 (71.5574, 34.1768) -> (71.5574, 35.2636)
  spline S101 degree 2 poles (71.5574, 35.2636) (71.8723, 35.418) (73.0024, 35.7206) (73.5087, 35.7206) knots 0 0 0 1 2 2 2
  spline S102 degree 2 poles (73.5087, 35.7206) (74.577, 35.7206) (75.7811, 34.5905) (75.7811, 33.6272) knots 0 0 0 1 2 2 2
  spline S103 degree 2 poles (75.7811, 33.6272) (75.7811, 33.1764) (75.5712, 32.4231) (75.3859, 32.102) knots 0 0 0 1 2 2 2
  spline S104 degree 2 poles (75.3859, 32.102) (75.2007, 31.7685) (74.6634, 31.114) (74.367, 30.799) knots 0 0 0 1 2 2 2
  spline S105 degree 2 poles (74.367, 30.799) (73.8854, 30.2742) (72.706, 29.1503) (72.354, 28.823) knots 0 0 0 1 2 2 2
  line L84 (72.354, 28.823) -> (76.0961, 28.823)
  line L85 (76.0961, 28.823) -> (76.0961, 27.94)
  point P0 (39.37, 0)
  dimension "d49" = 31.75
  constraints: 2 end point, 2 horizontal, 2 point on line
  measures "d49" distance between parallel lines of L1 L3
extrude "objectFileName" cut sketch "Sketch11" against normal blind 1.27
sketch "Sketch12" plane through (0, 0, 39.37) normal (0, 0, 1) x (1, 0, 0)
  line L0 (14.1055, 100.3659) -> (0, 101.6) projected
  line L1 (0, 0) -> (14.1055, 100.3659) projected
  line L2 (0, 101.6) -> (0, 0) projected
  line L3 (0, 101.6) -> (14.1055, 100.3659)
  line L4 (0, 0) -> (14.1055, 100.3659)
  line L5 (0, 101.6) -> (0, 0)
  constraints: 6 end point, 1 collinear
extrude "Extrusion11" add sketch "Sketch12" along normal blind 12.7
sketch "Sketch13" plane through (0, 0, -39.37) normal (0, 0, -1) x (-1, 0, 0)
  line L0 (0, 101.6) -> (-14.1055, 100.3659) projected
  line L1 (0, 0) -> (0, 101.6) projected
  line L2 (-14.1055, 100.3659) -> (0, 0) projected
  line L3 (0, 101.6) -> (0, 0) projected
  line L4 (-14.1055, 100.3659) -> (0, 101.6)
  line L5 (0, 101.6) -> (0, 0)
  line L6 (0, 0) -> (-14.1055, 100.3659)
  constraints: 6 end point, 1 collinear
extrude "Extrusion12" add sketch "Sketch13" along normal blind 7.9375
equation "\"d24\" = textDepth"
equation "\"d27\" = reliefHoleDepth"
equation "\"d42\" = textDepth"
equation "\"d50\" = textDepth"
equation "\"reliefHoleDepth\" = 6.35"
equation "\"textDepth\" = 1.27"
body "Solid1"
